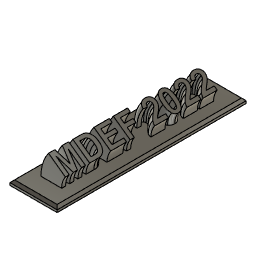
nameplate (Autodesk Fusion 360 design; units mm, degrees)
Autodesk Fusion 360 part; units mm, degrees
box "BoxPrimitive1" add length 200 width 50 height 5 placed x (0, 1, 0) y (-1, 0, 0) z (0, 0, 1) at (0, 0, 0)
sketch "Sketch2" plane through (0, 0, 5) normal (0, 0, 1) x (-1, 0, 0)
  line L0 (0, -200) -> (50, -200)
  line L1 (50, -200) -> (50, 0)
  line L2 (50, 0) -> (0, 0)
  line L3 (0, 0) -> (0, -200)
  line L4 (2.9104, -19.6517) -> (2.3415, -196.4739) construction
  line L5 (2.3415, -196.4739) -> (36.3332, -196.5833) construction
  line L6 (36.3332, -196.5833) -> (36.9021, -19.7611) construction
  line L7 (36.9021, -19.7611) -> (2.9104, -19.6517) construction
  dimension "d6" = 22
  text T0 "MDEF 2022" font "Arial" height 22 bold align left top in box 176.8231 x 33.9919 at (2.9104, -19.6517) x (-0.003218, -0.999995) y (0.999995, -0.003218) spacing 1 kerned
sketch "Sketch3" plane through (0, 0, 0) normal (0, -1, 0) x (1, 0, 0)
  line L0 (-50, 5) -> (-50, 0)
  line L1 (-50, 0) -> (0, 0)
  line L2 (0, 0) -> (0, 5)
  line L3 (0, 5) -> (-50, 5)
  arc A0 (3.0752, 10.4236) -> (0, 5) centre (6.3202, 5) ccw
  constraint tangent L2 A0
  constraint coincident L2.end L3.start
sweep "Sweep1" add profiles "Sketch2" path "Sketch3" along A0 for 0.6 of its length starting at (3.0752, 0, 10.4236) heading (-0.8581, 0, -0.5134) section 1 text T0
chamfer "Chamfer1" distance 2.5 angle 45 4 edges at (-50, 100, 5) (-25, 0, 5) (0, 100, 5) (-25, 200, 5)
